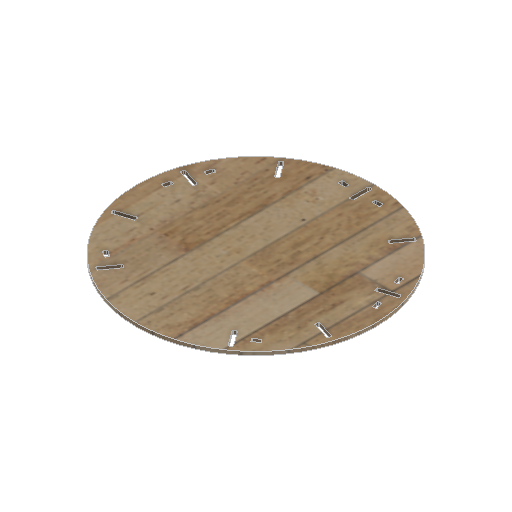
# Autodesk Inventor part: Base - A
Saved by Autodesk Inventor 2021 (Build 250183000, 183)
## iProperties
Created: 2020-03-07
Part Number: Base - A
Material: Wood (Maple)
Document SubType Name: Modeling
Designer: Daniel Wikman
Density: 0.67 g/cm^3
Appearance: Natural Maple - Glossy Dark Tint
Author: Daniel Wikman
Autodesk Inventor part; units mm, degrees
ref_plane "YZ Plane" through (0, 0, 0) normal (1, 0, 0) x (0, 1, 0)
ref_plane "XZ Plane" through (0, 0, 0) normal (0, 1, 0) x (-1, 0, 0)
ref_plane "XY Plane" through (0, 0, 0) normal (0, 0, 1) x (1, 0, 0)
sketch "Sketch2" plane through (0, 0, 0) normal (0, 1, 0) x (-1, 0, 0)
  circle A0 centre (0, 0) radius 200
  dimension "d9" = 400
  constraints: 1 centre point, 1 coincident
  measures "d9" diameter of A0
sketch "Sketch1" plane through (0, 0, 0) normal (0, 1, 0) x (-1, 0, 0)
  line L0 (1.9167, -191.4) -> (-1.9167, -191.4)
  line L1 (-3.25, -190.0667) -> (-3.25, -160.0667)
  line L2 (-1.9167, -158.7333) -> (1.9167, -158.7333)
  line L3 (3.25, -160.0667) -> (3.25, -190.0667)
  arc A0 (1.9167, -191.4) -> (3.25, -190.0667) centre (1.9167, -190.0667) ccw
  arc A1 (-3.25, -190.0667) -> (-1.9167, -191.4) centre (-1.9167, -190.0667) ccw
  arc A2 (-1.9167, -158.7333) -> (-3.25, -160.0667) centre (-1.9167, -160.0667) ccw
  arc A3 (3.25, -160.0667) -> (1.9167, -158.7333) centre (1.9167, -160.0667) ccw
  line L4 (114.0527, -153.7193) -> (110.9515, -155.9724)
  line L5 (109.0891, -155.6775) -> (91.4555, -131.407)
  line L6 (91.7505, -129.5446) -> (94.8517, -127.2914)
  line L7 (96.7141, -127.5864) -> (114.3477, -151.8569)
  arc A4 (114.0527, -153.7193) -> (114.3477, -151.8569) centre (113.269, -152.6406) ccw
  arc A5 (109.0891, -155.6775) -> (110.9515, -155.9724) centre (110.1678, -154.8938) ccw
  arc A6 (91.7505, -129.5446) -> (91.4555, -131.407) centre (92.5342, -130.6232) ccw
  arc A7 (96.7141, -127.5864) -> (94.8517, -127.2914) centre (95.6354, -128.3701) ccw
  line L8 (182.6245, -57.323) -> (181.4399, -60.9687)
  line L9 (179.7598, -61.8248) -> (151.2281, -52.5543)
  line L10 (150.3721, -50.8742) -> (151.5567, -47.2284)
  line L11 (153.2368, -46.3724) -> (181.7684, -55.6429)
  arc A8 (182.6245, -57.323) -> (181.7684, -55.6429) centre (181.3564, -56.911) ccw
  arc A9 (179.7598, -61.8248) -> (181.4399, -60.9687) centre (180.1719, -60.5567) ccw
  arc A10 (150.3721, -50.8742) -> (151.2281, -52.5543) centre (151.6402, -51.2862) ccw
  arc A11 (153.2368, -46.3724) -> (151.5567, -47.2284) centre (152.8247, -47.6405) ccw
  line L12 (181.4399, 60.9687) -> (182.6245, 57.323)
  line L13 (181.7684, 55.6429) -> (153.2368, 46.3724)
  line L14 (151.5567, 47.2284) -> (150.3721, 50.8742)
  line L15 (151.2281, 52.5543) -> (179.7598, 61.8248)
  arc A12 (181.4399, 60.9687) -> (179.7598, 61.8248) centre (180.1719, 60.5567) ccw
  arc A13 (181.7684, 55.6429) -> (182.6245, 57.323) centre (181.3564, 56.911) ccw
  arc A14 (151.5567, 47.2284) -> (153.2368, 46.3724) centre (152.8247, 47.6405) ccw
  arc A15 (151.2281, 52.5543) -> (150.3721, 50.8742) centre (151.6402, 51.2862) ccw
  line L16 (110.9515, 155.9724) -> (114.0527, 153.7193)
  line L17 (114.3477, 151.8569) -> (96.7141, 127.5864)
  line L18 (94.8517, 127.2914) -> (91.7505, 129.5446)
  line L19 (91.4555, 131.407) -> (109.0891, 155.6775)
  arc A16 (110.9515, 155.9724) -> (109.0891, 155.6775) centre (110.1678, 154.8938) ccw
  arc A17 (114.3477, 151.8569) -> (114.0527, 153.7193) centre (113.269, 152.6406) ccw
  arc A18 (94.8517, 127.2914) -> (96.7141, 127.5864) centre (95.6354, 128.3701) ccw
  arc A19 (91.4555, 131.407) -> (91.7505, 129.5446) centre (92.5342, 130.6232) ccw
  line L20 (-114.0527, 153.7193) -> (-110.9515, 155.9724)
  line L21 (-109.0891, 155.6775) -> (-91.4555, 131.407)
  line L22 (-91.7505, 129.5446) -> (-94.8517, 127.2914)
  line L23 (-96.7141, 127.5864) -> (-114.3477, 151.8569)
  arc A20 (-114.0527, 153.7193) -> (-114.3477, 151.8569) centre (-113.269, 152.6406) ccw
  arc A21 (-109.0891, 155.6775) -> (-110.9515, 155.9724) centre (-110.1678, 154.8938) ccw
  arc A22 (-91.7505, 129.5446) -> (-91.4555, 131.407) centre (-92.5342, 130.6232) ccw
  arc A23 (-96.7141, 127.5864) -> (-94.8517, 127.2914) centre (-95.6354, 128.3701) ccw
  line L24 (-182.6245, 57.323) -> (-181.4399, 60.9687)
  line L25 (-179.7598, 61.8248) -> (-151.2281, 52.5543)
  line L26 (-150.3721, 50.8742) -> (-151.5567, 47.2284)
  line L27 (-153.2368, 46.3724) -> (-181.7684, 55.6429)
  arc A24 (-182.6245, 57.323) -> (-181.7684, 55.6429) centre (-181.3564, 56.911) ccw
  arc A25 (-179.7598, 61.8248) -> (-181.4399, 60.9687) centre (-180.1719, 60.5567) ccw
  arc A26 (-150.3721, 50.8742) -> (-151.2281, 52.5543) centre (-151.6402, 51.2862) ccw
  arc A27 (-153.2368, 46.3724) -> (-151.5567, 47.2284) centre (-152.8247, 47.6405) ccw
  line L28 (-181.4399, -60.9687) -> (-182.6245, -57.323)
  line L29 (-181.7684, -55.6429) -> (-153.2368, -46.3724)
  line L30 (-151.5567, -47.2284) -> (-150.3721, -50.8742)
  line L31 (-151.2281, -52.5543) -> (-179.7598, -61.8248)
  arc A28 (-181.4399, -60.9687) -> (-179.7598, -61.8248) centre (-180.1719, -60.5567) ccw
  arc A29 (-181.7684, -55.6429) -> (-182.6245, -57.323) centre (-181.3564, -56.911) ccw
  arc A30 (-151.5567, -47.2284) -> (-153.2368, -46.3724) centre (-152.8247, -47.6405) ccw
  arc A31 (-151.2281, -52.5543) -> (-150.3721, -50.8742) centre (-151.6402, -51.2862) ccw
  line L32 (-110.9515, -155.9724) -> (-114.0527, -153.7193)
  line L33 (-114.3477, -151.8569) -> (-96.7141, -127.5864)
  line L34 (-94.8517, -127.2914) -> (-91.7505, -129.5446)
  line L35 (-91.4555, -131.407) -> (-109.0891, -155.6775)
  arc A32 (-110.9515, -155.9724) -> (-109.0891, -155.6775) centre (-110.1678, -154.8938) ccw
  arc A33 (-114.3477, -151.8569) -> (-114.0527, -153.7193) centre (-113.269, -152.6406) ccw
  arc A34 (-94.8517, -127.2914) -> (-96.7141, -127.5864) centre (-95.6354, -128.3701) ccw
  arc A35 (-91.4555, -131.407) -> (-91.7505, -129.5446) centre (-92.5342, -130.6232) ccw
  point P0 (0, 0)
  dimension "d2" = 6.5
  dimension "d3" = 1.3333
  dimension "d4" = 30
  dimension "d5" = 3.25
  constraints: 72 end point, 72 point on circle, 36 centre point, 8 tangent, 3 equal radius, 2 parallel, 1 horizontal, 1 perpendicular
  measures "d2" distance between parallel lines of L1 L3
  measures "d3" radius of A0
  measures "d4" distance of L1.start L1.end
  measures "d5" distance from line of point (0, 0) L1
extrude "Extrusion1" add sketch "Sketch2" along normal blind 6
extrude "Extrusion2" cut sketch "Sketch1" along normal through all
sketch "Sketch3" plane through (0, 6, 0) normal (0, 1, 0) x (1, 0, 0)
  line L0 (23.25, 178.3167) -> (33.25, 178.3167)
  line L1 (34.5833, 176.9833) -> (34.5833, 173.15)
  line L2 (33.25, 171.8167) -> (23.25, 171.8167)
  line L3 (21.9167, 173.15) -> (21.9167, 176.9833)
  line L4 (-1.9167, 191.4) -> (1.9167, 191.4) projected
  line L5 (1.9167, 158.7333) -> (-1.9167, 158.7333) projected
  line L6 (3.25, 160.0667) -> (3.25, 190.0667) projected
  arc A0 (23.25, 178.3167) -> (21.9167, 176.9833) centre (23.25, 176.9833) ccw
  arc A1 (33.25, 171.8167) -> (34.5833, 173.15) centre (33.25, 173.15) ccw
  arc A2 (34.5833, 176.9833) -> (33.25, 178.3167) centre (33.25, 176.9833) ccw
  arc A3 (21.9167, 173.15) -> (23.25, 171.8167) centre (23.25, 173.15) ccw
  line L7 (1.9167, 191.4) -> (-1.9167, 191.4) projected
  line L8 (0, 191.4) -> (0, 158.7333)
  line L9 (-1.9167, 158.7333) -> (1.9167, 158.7333) projected
  line L10 (-23.25, 178.3167) -> (-33.25, 178.3167)
  line L11 (-34.5833, 176.9833) -> (-34.5833, 173.15)
  line L12 (-33.25, 171.8167) -> (-23.25, 171.8167)
  line L13 (-21.9167, 173.15) -> (-21.9167, 176.9833)
  arc A4 (-21.9167, 176.9833) -> (-23.25, 178.3167) centre (-23.25, 176.9833) ccw
  arc A5 (-34.5833, 173.15) -> (-33.25, 171.8167) centre (-33.25, 173.15) ccw
  arc A6 (-33.25, 178.3167) -> (-34.5833, 176.9833) centre (-33.25, 176.9833) ccw
  arc A7 (-23.25, 171.8167) -> (-21.9167, 173.15) centre (-23.25, 173.15) ccw
  line L14 (3.25, 175.0667) -> (8.3501, 175.0667)
  line L15 (-162.4046, 77.2149) -> (-159.3144, 86.7255)
  line L16 (-157.6343, 87.5816) -> (-153.9886, 86.397)
  line L17 (-153.1325, 84.7169) -> (-156.2227, 75.2063)
  line L18 (-157.9028, 74.3503) -> (-161.5485, 75.5348)
  arc A8 (-162.4046, 77.2149) -> (-161.5485, 75.5348) centre (-161.1365, 76.8029) ccw
  arc A9 (-157.9028, 74.3503) -> (-156.2227, 75.2063) centre (-157.4908, 75.6184) ccw
  arc A10 (-153.1325, 84.7169) -> (-153.9886, 86.397) centre (-154.4006, 85.1289) ccw
  arc A11 (-157.6343, 87.5816) -> (-159.3144, 86.7255) centre (-158.0463, 86.3135) ccw
  line L19 (-171.4481, 32.6623) -> (-175.0938, 33.8469)
  arc A12 (-170.592, 30.9822) -> (-171.4481, 32.6623) centre (-171.8601, 31.3942) ccw
  arc A13 (-175.0938, 33.8469) -> (-176.7739, 32.9908) centre (-175.5058, 32.5788) ccw
  arc A14 (-179.864, 23.4803) -> (-179.008, 21.8002) centre (-178.596, 23.0682) ccw
  line L20 (-179.008, 21.8002) -> (-175.3623, 20.6156)
  arc A15 (-175.3623, 20.6156) -> (-173.6822, 21.4716) centre (-174.9503, 21.8837) ccw
  line L21 (-176.7739, 32.9908) -> (-179.864, 23.4803)
  line L22 (-173.6822, 21.4716) -> (-170.592, 30.9822)
  line L23 (-123.6216, -130.5952) -> (-131.7117, -124.7174)
  line L24 (-132.0067, -122.855) -> (-129.7535, -119.7537)
  line L25 (-127.8911, -119.4587) -> (-119.8009, -125.3366)
  line L26 (-119.506, -127.199) -> (-121.7591, -130.3002)
  arc A16 (-123.6216, -130.5952) -> (-121.7591, -130.3002) centre (-122.8378, -129.5165) ccw
  arc A17 (-119.506, -127.199) -> (-119.8009, -125.3366) centre (-120.5847, -126.4153) ccw
  arc A18 (-127.8911, -119.4587) -> (-129.7535, -119.7537) centre (-128.6748, -120.5374) ccw
  arc A19 (-132.0067, -122.855) -> (-131.7117, -124.7174) centre (-130.928, -123.6387) ccw
  line L27 (119.506, -127.199) -> (121.7591, -130.3002)
  arc A20 (119.8009, -125.3366) -> (119.506, -127.199) centre (120.5847, -126.4153) ccw
  arc A21 (121.7591, -130.3002) -> (123.6216, -130.5952) centre (122.8378, -129.5165) ccw
  arc A22 (131.7117, -124.7174) -> (132.0067, -122.855) centre (130.928, -123.6387) ccw
  line L28 (132.0067, -122.855) -> (129.7535, -119.7537)
  arc A23 (129.7535, -119.7537) -> (127.8911, -119.4587) centre (128.6748, -120.5374) ccw
  line L29 (123.6216, -130.5952) -> (131.7117, -124.7174)
  line L30 (127.8911, -119.4587) -> (119.8009, -125.3366)
  line L31 (176.7739, 32.9908) -> (179.864, 23.4803)
  line L32 (179.008, 21.8002) -> (175.3623, 20.6156)
  line L33 (173.6822, 21.4716) -> (170.592, 30.9822)
  line L34 (171.4481, 32.6623) -> (175.0938, 33.8469)
  arc A24 (176.7739, 32.9908) -> (175.0938, 33.8469) centre (175.5058, 32.5788) ccw
  arc A25 (171.4481, 32.6623) -> (170.592, 30.9822) centre (171.8601, 31.3942) ccw
  arc A26 (173.6822, 21.4716) -> (175.3623, 20.6156) centre (174.9503, 21.8837) ccw
  arc A27 (179.008, 21.8002) -> (179.864, 23.4803) centre (178.596, 23.0682) ccw
  line L35 (157.9028, 74.3503) -> (161.5485, 75.5348)
  arc A28 (156.2227, 75.2063) -> (157.9028, 74.3503) centre (157.4908, 75.6184) ccw
  arc A29 (161.5485, 75.5348) -> (162.4046, 77.2149) centre (161.1365, 76.8029) ccw
  arc A30 (159.3144, 86.7255) -> (157.6343, 87.5816) centre (158.0463, 86.3135) ccw
  line L36 (157.6343, 87.5816) -> (153.9886, 86.397)
  arc A31 (153.9886, 86.397) -> (153.1325, 84.7169) centre (154.4006, 85.1289) ccw
  line L37 (162.4046, 77.2149) -> (159.3144, 86.7255)
  line L38 (153.1325, 84.7169) -> (156.2227, 75.2063)
  point P0 (0, 0)
  dimension "d14" = 6.5
  dimension "d20" = 18.6667
  dimension "d21" = 1.3333
  dimension "d22" = 1.3333
  dimension "d36" = 32.6667
  dimension "d37" = 3.25
  dimension "d38" = 13.0833
  dimension "d39" = 13.0833
  dimension "d43" = 10
  constraints: 68 end point, 64 point on circle, 32 centre point, 12 symmetric about line, 8 tangent, 3 midpoint, 2 equal radius, 2 horizontal, 2 parallel, 1 perpendicular, 4 other
  measures "d14" distance between parallel lines of L2 L0
  measures "d20" distance between parallel lines of L6 L3
  measures "d21" radius of A0
  measures "d22" radius of A3
  measures "d36" distance of L8.end L8.start
  measures "d37" distance between parallel lines of L14 L2
  measures "d38" distance between parallel lines of L0 L4
  measures "d39" distance between parallel lines of L5 L2
  measures "d43" distance of L0.start L0.end
extrude "Extrusion3" cut sketch "Sketch3" against normal through all
body "Solid1"
